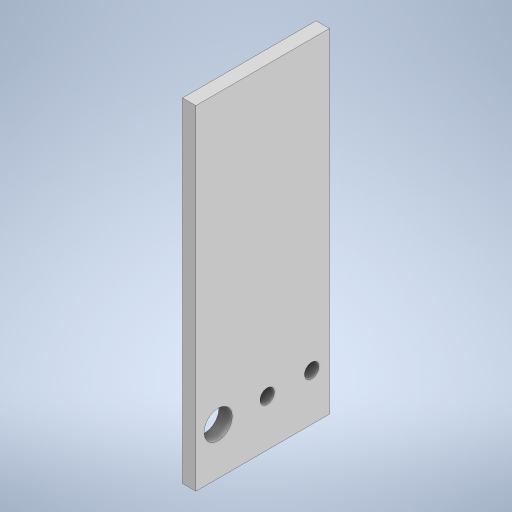
# Autodesk Inventor part: Side_Plate1
Saved by Autodesk Inventor 2023 (Build 270158000, 158)
## iProperties
Created: 2023-02-10
Part Number: Side_Plate1
Material: Generic
Document SubType Name: Modeling
Designer: deepa
Density: 1 g/cm^3
Appearance: Default
Author: deepa
Autodesk Inventor part; units mm, degrees
ref_plane "YZ Plane" through (0, 0, 0) normal (1, 0, 0) x (0, 1, 0)
ref_plane "XZ Plane" through (0, 0, 0) normal (0, 1, 0) x (-1, 0, 0)
ref_plane "XY Plane" through (0, 0, 0) normal (0, 0, 1) x (1, 0, 0)
sketch "Sketch1" plane through (0, 0, 0) normal (1, 0, 0) x (0, 1, 0)
  point P0 (0, 0)
sketch "Sketch2" plane through (0, 0, 0) normal (1, 0, 0) x (0, 1, 0)
  line L0 (72.7327, -29.8637) -> (-77.2673, -29.8637)
  line L1 (-77.2673, -29.8637) -> (-77.2673, 30.1363)
  line L2 (-77.2673, 30.1363) -> (72.7327, 30.1363)
  line L3 (72.7327, 30.1363) -> (72.7327, -29.8637)
  point P0 (0, 0)
  dimension "d0" = 150
  dimension "d1" = 60
  constraints: 8 end point, 2 parallel, 1 horizontal, 1 perpendicular
  measures "d0" distance of L1.end L2.end
  measures "d1" distance of L0.end L1.end
extrude "Extrusion1" add sketch "Sketch2" along normal blind 6
sketch "Sketch3" plane through (6, 0, 0) normal (1, 0, 0) x (0, 0, -1)
  line L0 (-26.5033, -56.2673) -> (30.2307, -56.2673) construction
  line L1 (-30.1363, -77.2673) -> (29.8637, -77.2673) projected
  circle A0 centre (21.8637, -56.2673) radius 3.25
  circle A1 centre (1.8637, -56.2673) radius 3.25
  circle A2 centre (-20.1363, -56.2673) radius 6.35
  line L2 (29.8637, -77.2673) -> (29.8637, 72.7327) projected
  line L3 (-30.1363, 72.7327) -> (-30.1363, -77.2673) projected
  point P0 (0, 0)
  dimension "d4" = 21
  dimension "d5" = 6.5
  dimension "d6" = 6.5
  dimension "d7" = 12.7
  dimension "d8" = 8
  dimension "d9" = 20
  dimension "d10" = 10
  constraints: 3 centre point, 2 end point, 2 point on line, 1 horizontal, 1 midpoint
  measures "d4" distance between parallel lines of L0 L1
  measures "d5" diameter of A0
  measures "d6" diameter of A1
  measures "d7" diameter of A2
  measures "d8" distance from line of L2 A0.centre
  measures "d9" distance of A1.centre A0.centre
  measures "d10" distance from line of L3 A2.centre
extrude "Extrusion2" cut sketch "Sketch3" against normal blind 6
body "Solid1"
